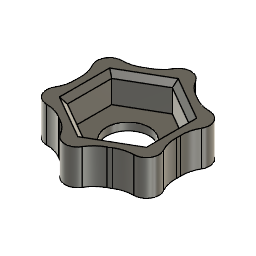
OpenATC-ER20-A-Nut-holder (Autodesk Fusion 360 design; units mm, degrees)
Autodesk Fusion 360 part; units mm, degrees
sketch "Sketch1" plane through (0, 0, 0) normal (0, 0, 1) x (1, 0, 0)
  circle A0 centre (0, 0) radius 8.5
  circle A1 centre (0, 0) radius 20
  dimension "d1" = 17
  dimension "d2" = 40
  constraint coincident A0.centre A1.centre
  measures "d1" diameter of A0
  measures "d2" diameter of A1
extrude "Extrude1" add sketch "Sketch1" along normal blind 14
sketch "Sketch2" plane through (0, 0, 14) normal (0, 0, 1) x (-1, 0, 0)
  circle A0 centre (0, 0) radius 8.5
  circle A1 centre (0, 0) radius 20
  line L0 (-15.25, -8.8046) -> (0, -17.6092)
  line L1 (0, -17.6092) -> (15.25, -8.8046)
  line L2 (15.25, -8.8046) -> (15.25, 8.8046)
  line L3 (15.25, 8.8046) -> (0, 17.6092)
  line L4 (0, 17.6092) -> (-15.25, 8.8046)
  line L5 (-15.25, 8.8046) -> (-15.25, -8.8046)
  line L6 (0, 0) -> (0, -24.7489) construction
  dimension "d5" = 15.25
  constraint coincident A0.centre A1.centre
  constraint vertical L6
  constraint coincident L0.end L6
  measures "d5" distance of A0.centre L5
extrude "Extrude2" cut sketch "Sketch2" against normal blind 11 contours L0 L1 L2 L3 L4 L5
sketch "Sketch3" plane through (0, 0, 14) normal (0, 0, 1) x (-1, 0, 0)
  line L0 (0, -17.6092) -> (-15.25, -8.8046)
  line L1 (-15.25, -8.8046) -> (-15.25, 8.8046)
  line L2 (-15.25, 8.8046) -> (0, 17.6092)
  line L3 (0, 17.6092) -> (15.25, 8.8046)
  line L4 (15.25, 8.8046) -> (15.25, -8.8046)
  line L5 (15.25, -8.8046) -> (0, -17.6092)
  circle A0 centre (0, 0) radius 20
  line L6 (0, -20) -> (0, 20) construction
  line L7 (20, 0) -> (-20, 0) construction
  arc A1 (-4.3301, -22.5) -> (4.3301, -22.5) centre (0, -20) ccw
  line L8 (0, -20) -> (0, -25) construction
  line L9 (0, -20) -> (4.3301, -22.5) construction
  line L10 (0, -20) -> (-4.3301, -22.5) construction
  arc A2 (9.3264, -17.6923) -> (4.3301, -22.5) centre (15.1554, -28.75) ccw
  arc A3 (-4.3301, -22.5) -> (-9.3264, -17.6923) centre (-15.1554, -28.75) ccw
  arc A4 (-9.3264, -17.6923) -> (9.3264, -17.6923) centre (0, 0) ccw
  arc A5 (17.3205, -15) -> (21.6506, -7.5) centre (17.3205, -10) ccw
  arc A6 (17.3205, -15) -> (10.6588, -16.9231) centre (17.3205, -27.5) ccw
  arc A7 (10.6588, -16.9231) -> (19.9852, -0.7692) centre (0, 0) ccw
  arc A8 (19.9852, -0.7692) -> (21.6506, -7.5) centre (32.476, -1.25) ccw
  arc A9 (21.6506, 7.5) -> (17.3205, 15) centre (17.3205, 10) ccw
  arc A10 (21.6506, 7.5) -> (19.9852, 0.7692) centre (32.476, 1.25) ccw
  arc A11 (19.9852, 0.7692) -> (10.6588, 16.9231) centre (0, 0) ccw
  arc A12 (10.6588, 16.9231) -> (17.3205, 15) centre (17.3205, 27.5) ccw
  arc A13 (4.3301, 22.5) -> (-4.3301, 22.5) centre (0, 20) ccw
  arc A14 (4.3301, 22.5) -> (9.3264, 17.6923) centre (15.1554, 28.75) ccw
  arc A15 (9.3264, 17.6923) -> (-9.3264, 17.6923) centre (0, 0) ccw
  arc A16 (-9.3264, 17.6923) -> (-4.3301, 22.5) centre (-15.1554, 28.75) ccw
  arc A17 (-17.3205, 15) -> (-21.6506, 7.5) centre (-17.3205, 10) ccw
  arc A18 (-17.3205, 15) -> (-10.6588, 16.9231) centre (-17.3205, 27.5) ccw
  arc A19 (-10.6588, 16.9231) -> (-19.9852, 0.7692) centre (0, 0) ccw
  arc A20 (-19.9852, 0.7692) -> (-21.6506, 7.5) centre (-32.476, 1.25) ccw
  arc A21 (-21.6506, -7.5) -> (-17.3205, -15) centre (-17.3205, -10) ccw
  arc A22 (-21.6506, -7.5) -> (-19.9852, -0.7692) centre (-32.476, -1.25) ccw
  arc A23 (-19.9852, -0.7692) -> (-10.6588, -16.9231) centre (0, 0) ccw
  arc A24 (-10.6588, -16.9231) -> (-17.3205, -15) centre (-17.3205, -27.5) ccw
  dimension "d10" = 60
  dimension "d11" = 60
  dimension "d12" = 5
  dimension "d14" = 360
  constraint coincident A0 L6.start
  constraint coincident A0 L6.end
  constraint vertical L6
  constraint coincident A0 L7.start
  constraint coincident A0 L7.end
  constraint perpendicular L6 L7
  constraint coincident A0.centre L6
  constraint coincident A0.centre L7
  constraint parallel L6 L8
  constraint coincident L6.start A1.centre
  constraint tangent A0 A2
  constraint coincident A0 A2.start
  constraint tangent A1 A2
  constraint tangent A0 A3
  constraint coincident A0 A3.end
  constraint tangent A1 A3
  constraint coincident A1 L8.end
  constraint coincident L6.start A4
  measures "d10" angle of L8 L10
  measures "d11" angle of L8 L9
  measures "d12" radius of A1
extrude "Extrude3" add sketch "Sketch3" against normal up to surface (14 mm away) contours A0 A9 A10 A11 A12 | A0 A5 A6 A7 A8 | A0 A13 A14 A15 A16 | A0 A1 A2 A3 A4 | A0 A17 A18 A19 A20 | A0 A21 A22 A23 A24
chamfer "Chamfer1" distance 2 angle 45 6 edges at (-7.625, 13.2069, 14) (-15.25, 0, 14) (-7.625, -13.2069, 14) (7.625, -13.2069, 14) (15.25, 0, 14) (7.625, 13.2069, 14)
sketch "Sketch4" plane through (0, 0, 0) normal (0, 0, -1) x (1, 0, 0)
  circle A0 centre (0, 0) radius 8.5
  arc A1 (-9.3264, 17.6923) -> (-10.6588, 16.9231) centre (0, 0) ccw
  arc A2 (-17.3205, 15) -> (-10.6588, 16.9231) centre (-17.3205, 27.5) ccw
  arc A3 (-17.3205, 15) -> (-21.6506, 7.5) centre (-17.3205, 10) ccw
  arc A4 (-19.9852, 0.7692) -> (-21.6506, 7.5) centre (-32.476, 1.25) ccw
  arc A5 (-19.9852, 0.7692) -> (-19.9852, -0.7692) centre (0, 0) ccw
  arc A6 (-21.6506, -7.5) -> (-19.9852, -0.7692) centre (-32.476, -1.25) ccw
  arc A7 (-21.6506, -7.5) -> (-17.3205, -15) centre (-17.3205, -10) ccw
  arc A8 (-10.6588, -16.9231) -> (-17.3205, -15) centre (-17.3205, -27.5) ccw
  arc A9 (-10.6588, -16.9231) -> (-9.3264, -17.6923) centre (0, 0) ccw
  arc A10 (-4.3301, -22.5) -> (-9.3264, -17.6923) centre (-15.1554, -28.75) ccw
  arc A11 (-4.3301, -22.5) -> (4.3301, -22.5) centre (0, -20) ccw
  arc A12 (9.3264, -17.6923) -> (4.3301, -22.5) centre (15.1554, -28.75) ccw
  arc A13 (9.3264, -17.6923) -> (10.6588, -16.9231) centre (0, 0) ccw
  arc A14 (17.3205, -15) -> (10.6588, -16.9231) centre (17.3205, -27.5) ccw
  arc A15 (17.3205, -15) -> (21.6506, -7.5) centre (17.3205, -10) ccw
  arc A16 (19.9852, -0.7692) -> (21.6506, -7.5) centre (32.476, -1.25) ccw
  arc A17 (19.9852, -0.7692) -> (19.9852, 0.7692) centre (0, 0) ccw
  arc A18 (21.6506, 7.5) -> (19.9852, 0.7692) centre (32.476, 1.25) ccw
  arc A19 (21.6506, 7.5) -> (17.3205, 15) centre (17.3205, 10) ccw
  arc A20 (10.6588, 16.9231) -> (17.3205, 15) centre (17.3205, 27.5) ccw
  arc A21 (10.6588, 16.9231) -> (9.3264, 17.6923) centre (0, 0) ccw
  arc A22 (4.3301, 22.5) -> (9.3264, 17.6923) centre (15.1554, 28.75) ccw
  arc A23 (4.3301, 22.5) -> (-4.3301, 22.5) centre (0, 20) ccw
  arc A24 (-9.3264, 17.6923) -> (-4.3301, 22.5) centre (-15.1554, 28.75) ccw
  circle A25 centre (0, 0) radius 13.25
  circle A26 centre (0, 0) radius 15.75
  dimension "d18" = 26.5
  dimension "d19" = 31.5
  constraint coincident A0.centre A1.centre
  constraint concentric A0 A26
  measures "d18" diameter of A25
  measures "d19" diameter of A26
extrude "Extrude4" cut sketch "Sketch4" against normal blind 1 contours A26
equation "d11 = d10"
